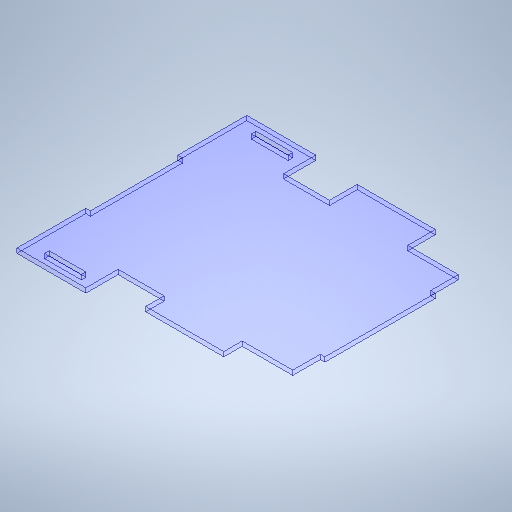
# Autodesk Inventor part: hood
Saved by Autodesk Inventor 2025.3 (Build 293356030, 356C)
## iProperties
Created: 2026-06-26
Part Number: hood
Material: Generic
Document SubType Name: Modeling
Designer: user
Density: 1 g/cm^3
Appearance: Blue
Author: user
Autodesk Inventor part; units mm, degrees
ref_plane "YZ Plane" through (0, 0, 0) normal (1, 0, 0) x (0, 1, 0)
ref_plane "XZ Plane" through (0, 0, 0) normal (0, 1, 0) x (-1, 0, 0)
ref_plane "XY Plane" through (0, 0, 0) normal (0, 0, 1) x (1, 0, 0)
sketch "Sketch1" plane through (0, 0, 0) normal (0, 1, 0) x (-1, 0, 0)
  line L0 (0, 0) -> (-75, 0)
  line L1 (-75, 0) -> (-75, -250)
  line L2 (-75, -250) -> (0, -250)
  line L3 (0, -250) -> (0, 0)
  line L4 (-20, -10) -> (-60, -10)
  line L5 (-60, -10) -> (-60, -15)
  line L6 (-60, -15) -> (-20, -15)
  line L7 (-20, -15) -> (-20, -10)
  line L8 (-75, -125) -> (0, -125) construction
  line L9 (-20, -240) -> (-60, -240)
  line L10 (-60, -240) -> (-60, -235)
  line L11 (-60, -235) -> (-20, -235)
  line L12 (-20, -235) -> (-20, -240)
  line L13 (-75, -35) -> (-265, -35)
  line L14 (-265, -35) -> (-265, -215)
  line L15 (-265, -215) -> (-75, -215)
  line L16 (-75, -215) -> (-75, -35)
  line L17 (-265, -65) -> (-270, -65)
  line L18 (-270, -65) -> (-270, -185)
  line L19 (-270, -185) -> (-265, -185)
  line L20 (-265, -185) -> (-265, -65)
  line L21 (0, -75) -> (-5, -75)
  line L22 (-5, -75) -> (-5, -175)
  line L23 (-5, -175) -> (0, -175)
  line L24 (0, -175) -> (0, -75)
  line L25 (-125, -35) -> (-210, -35)
  line L26 (-210, -35) -> (-210, -15)
  line L27 (-210, -15) -> (-125, -15)
  line L28 (-125, -15) -> (-125, -35)
  line L29 (-125, -215) -> (-210, -215)
  line L30 (-210, -215) -> (-210, -245)
  line L31 (-210, -245) -> (-125, -245)
  line L32 (-125, -245) -> (-125, -215)
  point P0 (-75, -215)
  point P1 (-265, -185)
  point P2 (0, -175)
  dimension "d0" = 75
  dimension "d2" = 40
  dimension "d3" = 5
  dimension "d6" = 190
  dimension "d7" = 180
  dimension "d8" = 5
  dimension "d9" = 120
  dimension "d11" = 20
  dimension "d12" = 5
  dimension "d13" = 100
  dimension "d14" = 75
  dimension "d15" = 85
  dimension "d16" = 50
  dimension "d17" = 10
  dimension "d18" = 30
  dimension "d19" = 230
  dimension "d20" = 35
  constraints: 66 end point, 14 parallel, 7 horizontal, 7 perpendicular, 5 point on line, 4 symmetric about line, 2 midpoint
  measures "d0" distance of L2.end L1.end
  measures "d2" distance of L6.end L5.end
  measures "d3" distance of L5.end L4.end
  measures "d6" distance of L15.end L14.end
  measures "d7" distance of L14.end L13.end
  measures "d8" distance of L19.end L18.end
  measures "d9" distance of L18.end L17.end
  measures "d11" distance between parallel lines of L12 L3
  measures "d12" distance of L23.end L22.end
  measures "d13" distance of L22.end L21.end
  measures "d14" distance of L2.end L23.end
  measures "d15" distance of L26.end L27.end
  measures "d16" distance between parallel lines of L28 L1
  measures "d17" distance between parallel lines of L0 L4
  measures "d18" distance between parallel lines of L19 L15
  measures "d19" distance between parallel lines of L4 L9
  measures "d20" distance of L15.end L1.end
extrude "Extrusion1" add sketch "Sketch1" along normal blind 5 contours L3 L21 L22 L23 L2 L1 L0 | L1 L15 L14 L13 | L13 L26 L27 L28 | L32 L31 L30 L15 | L14 L19 L18 L17
body "Solid1"
